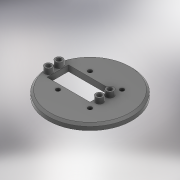
# Autodesk Inventor part: Gripper_Halter
Saved by Autodesk Inventor 2022 (Build 260153000, 153)
## iProperties
Created: 2023-07-17
Part Number: Gripper_Halter
Material: Generisch
Document SubType Name: Modeling
Designer: Alsaady
Density: 1 g/cm^3
Appearance: Glatt - Schwarz
Author: Alsaady
## iProperties of the stored document _3D-Druck.ipt
Created: 2023-07-17
Part Number: _3D-Druck
Material: Generisch
Document SubType Name: Modeling
Designer: Alsaady
Density: 1 g/cm^3
Appearance: Vorgabe
Author: Alsaady
Autodesk Inventor part; units mm, degrees
ref_plane "YZ Plane" through (0, 0, 0) normal (1, 0, 0) x (0, 1, 0)
ref_plane "XZ Plane" through (0, 0, 0) normal (0, 1, 0) x (-1, 0, 0)
ref_plane "XY Plane" through (0, 0, 0) normal (0, 0, 1) x (1, 0, 0)
sketch "Skizze1" plane through (0, 0, 0) normal (0, 1, 0) x (-1, 0, 0)
  circle A0 centre (0, 0) radius 40
  line L0 (15.25, 15.25) -> (-15.25, 15.25)
  line L1 (-15.25, 15.25) -> (-15.25, -15.25)
  line L2 (-15.25, -15.25) -> (15.25, -15.25)
  line L3 (15.25, -15.25) -> (15.25, 15.25)
  line L4 (0, -56) -> (0, 56) projected
  line L5 (56, 0) -> (-56, 0) projected
  circle A1 centre (15.25, 15.25) radius 2
  circle A2 centre (15.25, -15.25) radius 2
  circle A3 centre (-15.25, -15.25) radius 2
  circle A4 centre (-15.25, 15.25) radius 2
  point P0 (0, -15.25)
  point P1 (15.25, 0)
  dimension "d0" = 30.5
  dimension "d1" = 4
  dimension "d2" = 80
  constraints: 8 end point, 5 centre point, 5 coincident, 3 equal radius, 2 midpoint, 2 parallel, 2 perpendicular, 2 point on line, 1 horizontal
  measures "d0" distance of L2.end L0.start
  measures "d1" diameter of A1
  measures "d2" diameter of A0
extrude "Extrusion1" add sketch "Skizze1" along normal blind 5.5 contours L5 L3 A1 L0 L4 A0 | A0 L4 L2 A2 L3 L5 | L4 L0 A4 L1 L5 A0 | A0 L5 L1 A3 L2 L4 | L5 L4 L0 A1 L3 | L3 A2 L2 L4 L5 | L4 L5 L1 A4 L0 | L2 A3 L1 L5 L4
sketch "Skizze2" plane through (0, 5.5, 0) normal (0, 1, 0) x (1, 0, 0)
  line L0 (-11.75, -8.5) -> (11.75, -8.5)
  line L1 (11.75, -8.5) -> (11.75, 8.5)
  line L2 (11.75, 8.5) -> (-11.75, 8.5)
  line L3 (-11.75, 8.5) -> (-11.75, -8.5)
  line L4 (-56, 0) -> (56, 0) projected
  line L5 (0, 56) -> (0, -56) projected
  line L6 (-0.25, -8.5) -> (6.25, -8.5)
  line L7 (6.25, -8.5) -> (6.25, -5.2)
  line L8 (6.25, -5.2) -> (-0.25, -5.2)
  line L9 (-0.25, -5.2) -> (-0.25, -8.5)
  line L10 (-11.75, 8.5) -> (6.25, 8.5)
  line L11 (6.25, 8.5) -> (6.25, 5.2)
  line L12 (6.25, 5.2) -> (-11.75, 5.2)
  line L13 (-11.75, 5.2) -> (-11.75, 8.5)
  line L14 (-5.75, -8.5) -> (-5.75, 5.2) construction
  circle A0 centre (-5.75, -1.65) radius 1.75
  point P0 (0, 0)
  point P1 (-11.75, 0)
  point P2 (0, -8.5)
  point P3 (-11.75, 5.2)
  dimension "d5" = 23.5
  dimension "d6" = 17
  dimension "d7" = 12
  dimension "d8" = 5.5
  dimension "d9" = 3.3
  dimension "d10" = 3.3
  dimension "d11" = 5.5
  dimension "d12" = 3.5
  dimension "d17" = 6
  constraints: 26 end point, 6 parallel, 5 point on line, 4 perpendicular, 3 horizontal, 3 midpoint, 1 centre point
  measures "d5" distance of L1.end L2.end
  measures "d6" distance of L0.end L1.end
  measures "d7" distance from line of L1 L8.end
  measures "d8" distance between parallel lines of L1 L7
  measures "d9" distance of L8.end L6.start
  measures "d10" distance of L10.end L11.end
  measures "d11" distance from line of L11 L1.end
  measures "d12" diameter of A0
  measures "d17" distance between parallel lines of L3 L14
extrude "Extrusion2" [suppressed]
extrude "Extrusion3" [suppressed]
fillet "Rundung1" [suppressed]
fillet "Rundung2" [suppressed]
sketch "Skizze3" plane through (0, 5.5, 0) normal (0, 1, 0) x (1, 0, 0)
  line L0 (-30.75, -10.25) -> (10.25, -10.25)
  line L1 (10.25, -10.25) -> (10.25, 10.25)
  line L2 (10.25, 10.25) -> (-30.75, 10.25)
  line L3 (-30.75, 10.25) -> (-30.75, -10.25)
  line L4 (0, -10.25) -> (0, 10.25)
  circle A0 centre (-34.5, -5) radius 2.15
  circle A1 centre (-34.5, 5) radius 2.15
  circle A2 centre (14, 5) radius 2.15
  circle A3 centre (14, -5) radius 2.15
  line L5 (-10.25, -10.25) -> (-10.25, 10.25)
  line L6 (-56, 0) -> (56, 0) projected
  point P0 (0, 0)
  point P1 (0, 0)
  point P2 (-30.75, 0)
  point P3 (-10.25, 0)
  point P4 (10.25, 0)
  dimension "d20" = 48.5
  dimension "d21" = 4.3
  dimension "d22" = 20.5
  dimension "d23" = 41
  dimension "d24" = 34.5
  dimension "d25" = 10
  dimension "d35" = 10.25
  constraints: 12 end point, 4 centre point, 4 symmetric about line, 3 equal radius, 3 midpoint, 2 parallel, 2 perpendicular, 2 point on line, 1 coincident, 1 horizontal
  measures "d20" distance of A2.centre A1.centre
  measures "d21" diameter of A0
  measures "d22" distance of L0.end L1.end
  measures "d23" distance of L0.start L0.end
  measures "d24" horizontal distance of L4.start A0.centre
  measures "d25" distance of A2.centre A3.centre
  measures "d35" distance from line of point (0, 0) L5
extrude "Extrusion4" cut sketch "Skizze3" against normal through all
fillet "Rundung3" radius 2 4 edges at (-36.65, 0, 5) (-36.65, 0, -5) (11.85, 0, 5) (11.85, 0, -5)
sketch "Skizze4" plane through (0, 5.5, 0) normal (0, 1, 0) x (1, 0, 0)
  circle A0 centre (14, -5) radius 2.15 projected
  circle A1 centre (14, 5) radius 2.15 projected
  circle A2 centre (-34.5, 5) radius 2.15 projected
  circle A3 centre (-34.5, -5) radius 2.15 projected
  circle A4 centre (-34.5, -5) radius 3.5
  circle A5 centre (-34.5, 5) radius 3.5
  circle A6 centre (14, 5) radius 3.5
  circle A7 centre (14, -5) radius 3.5
  point P0 (0, 0)
  dimension "d29" = 7
  constraints: 4 centre point, 4 coincident, 3 equal radius
  measures "d29" diameter of A7
extrude "Extrusion5" add sketch "Skizze4" along normal blind 5
chamfer "Fase1" distance 2 angle 45 1 edges at (40, 5.5, 0)
equation "\"d8\" = d11"
equation "\"d9\" = d10"
